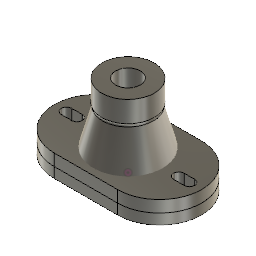
_4&#47;16&#47;19.19b655a6-d3a3-4cc6-afa9-02d68b133b6b (Autodesk Fusion 360 design; units mm, degrees)
Autodesk Fusion 360 part; units mm, degrees
note: some values were not read from the file. Set by a fixed rule: which face or edge a step refers to.
sketch "Sketch1" plane through (0, 0, 0) normal (0, 0, 1) x (1, 0, 0)
  line L0 (27, -36) -> (-27, -36)
  line L1 (-27, 36) -> (27, 36)
  arc A0 (-27, 36) -> (-27, -36) centre (-27, 0) ccw
  arc A1 (27, -36) -> (27, 36) centre (27, 0) ccw
  constraint parallel L0 L1
  constraint horizontal L0
  constraint tangent L1 A0
extrude "Extrude1" add sketch "Sketch1" along normal blind 9 makes body 1
sketch "Sketch2" plane through (0, 0, 9) normal (0, 0, 1) x (-1, 0, 0)
  arc A0 (27, -36) -> (27, 36) centre (27, 0) ccw
  line L0 (27, 36) -> (-27, 36)
  arc A1 (-27, 36) -> (-27, -36) centre (-27, 0) ccw
  line L1 (-27, -36) -> (27, -36)
  line L2 (43.5, -4.5) -> (52.5, -4.5)
  line L3 (52.5, 4.5) -> (43.5, 4.5)
  arc A2 (52.5, -4.5) -> (52.5, 4.5) centre (52.5, 0) ccw
  arc A3 (43.5, 4.5) -> (43.5, -4.5) centre (43.5, 0) ccw
  point P0 (48, 0)
  constraint parallel L2 L3
  constraint horizontal L2
extrude "Extrude2" cut sketch "Sketch2" against normal blind 53 contours L2 L3 A2 A3 bodies 1
sketch "Sketch3" plane through (0, 0, 9) normal (0, 0, 1) x (-1, 0, 0)
  line L0 (52.5, -4.5) -> (43.5, -4.5)
  arc A0 (43.5, 4.5) -> (43.5, -4.5) centre (43.5, 0) ccw
  line L1 (43.5, 4.5) -> (52.5, 4.5)
  arc A1 (52.5, -4.5) -> (52.5, 4.5) centre (52.5, 0) ccw
  arc A2 (27, -36) -> (27, 36) centre (27, 0) ccw
  line L2 (27, 36) -> (-27, 36)
  arc A3 (-27, 36) -> (-27, -36) centre (-27, 0) ccw
  line L3 (-27, -36) -> (27, -36)
  line L4 (-52.5, 4.5) -> (-43.5, 4.5)
  line L5 (-39, 0.0028) -> (-39, -0.0028)
  line L6 (-43.4972, -4.5) -> (-52.5, -4.5)
  arc A4 (-43.5028, -4.5) -> (-43.5, 4.5) centre (-43.5, 0) ccw
  arc A5 (-52.5, 4.5) -> (-52.5, -4.5) centre (-52.5, 0) ccw
  constraint perpendicular L4 L5
  constraint parallel L4 L6
  constraint horizontal L4
  constraint coincident L6 A4.start
  constraint coincident A4 L5.end
  constraint coincident A4 L6.start
  constraint coincident A4 L5.start
extrude "Extrude3" cut sketch "Sketch3" against normal blind 31 contours L4 L5 L6 A4 A5 bodies 1
copy_body "Body->Comp1" bodies 1 removing the originals makes body 2 in component "Component"
sketch "Sketch4" plane through (0, 0, 0) normal (0, 1, 0) x (1, 0, 0)
sketch "Sketch5" plane through (0, 0, 9) normal (0, 0, 1) x (-1, 0, 0)
  line L0 (-52.5, 4.5) -> (-43.5, 4.5)
  arc A0 (-43.5028, -4.5) -> (-43.5, 4.5) centre (-43.5, 0) ccw
  line L1 (-43.5028, -4.5) -> (-52.5, -4.5)
  arc A1 (-52.5, 4.5) -> (-52.5, -4.5) centre (-52.5, 0) ccw
  line L2 (52.5, -4.5) -> (43.5, -4.5)
  arc A2 (43.5, 4.5) -> (43.5, -4.5) centre (43.5, 0) ccw
  line L3 (43.5, 4.5) -> (52.5, 4.5)
  arc A3 (52.5, -4.5) -> (52.5, 4.5) centre (52.5, 0) ccw
  arc A4 (27, -36) -> (27, 36) centre (27, 0) ccw
  line L4 (27, 36) -> (-27, 36)
  arc A5 (-27, 36) -> (-27, -36) centre (-27, 0) ccw
  line L5 (-27, -36) -> (27, -36)
sketch "Sketch6" plane through (0, 0, 0) normal (0, 1, 0) x (1, 0, 0)
  line L0 (-63, -9) -> (-27, -9)
  line L1 (0, -9) -> (-33, -9)
  line L2 (0, -9) -> (0, -52)
  line L3 (0, -52) -> (-21, -52)
  line L4 (-21, -52) -> (-33, -9)
  point P0 (0, -9)
  constraint coincident P0 L1.start
  constraint parallel L0 L1
  constraint perpendicular L1 L2
  constraint perpendicular L2 L3
revolve "Revolve1" add sketch "Sketch6" angle 360 about axis through (0, 0, 9) along (0, 0, 1) bodies 2 in component "Component"
sketch "Sketch7" plane through (0, 0, 0) normal (0, 1, 0) x (1, 0, 0)
  line L0 (27, 0) -> (-27, 0)
  line L1 (0, 0) -> (0, -47)
  line L2 (0, 0) -> (-30, 0)
  line L3 (0, -47) -> (-14.4884, -47)
  line L4 (-27, 0) -> (-14.4884, -47)
  dimension "d27" = 47
  dimension "d28" = 30
  constraint coincident L1.start L2.start
  constraint perpendicular L0 L1
  constraint perpendicular L1 L2
  constraint perpendicular L1 L3
  constraint coincident L0.end L4.start
  constraint coincident L3 L4.end
  measures "d27" distance of L1.start L1.end
  measures "d28" distance of L1.start L2.end
revolve "Revolve2" cut sketch "Sketch7" angle 360 about axis through (0, 0, 0) along (0, 0, 1) bodies 2 in component "Component"
sketch "Sketch8" plane through (0, 0, 52) normal (0, 0, 1) x (-1, 0, 0)
  circle A0 centre (0, 0) radius 21
  circle A1 centre (0, 0) radius 22.5
  dimension "d30" = 45
  constraint concentric A0 A1
  measures "d30" diameter of A1
extrude "Extrude1'" add sketch "Sketch8" along normal blind 18 contours A0 | A1 bodies 2 in component "Component"
sketch "Sketch9" plane through (0, 0, 70) normal (0, 0, 1) x (-1, 0, 0)
  circle A0 centre (0, 0) radius 22.5
  circle A1 centre (0, 0) radius 10.5
  dimension "d33" = 21
  constraint concentric A0 A1
  measures "d33" diameter of A1
extrude "Extrude2'" cut sketch "Sketch9" against normal blind 42 contours A1 bodies 2 in component "Component"
fillet "Fillet1" radius 3 1 edges at (-19.5789, 7.5939, 52) on bodies 2 in component "Component"
fillet "Fillet2" radius 3 1 edges at (30.7668, -11.9333, 9) on bodies 2 in component "Component"
sketch "Sketch10" plane through (0, 0, 9) normal (0, 0, 1) x (-1, 0, 0)
  circle A0 centre (0, 0) radius 16
  dimension "d38" = 32
  constraint coincident A0.centre origin
  measures "d38" diameter of A0
extrude "Extrude4" add sketch "Sketch10" along normal mid plane 24 separate body makes body 3
sketch "Sketch11" plane through (0, 0, 0) normal (0, 1, 0) x (1, 0, 0)
  line L0 (16, 3) -> (-16, 3)
  line L1 (0, 3) -> (-37, 3)
  line L2 (0, 3) -> (0, -51)
  line L3 (-44, -61) -> (-44, -51)
  line L4 (-30, -51) -> (-30, -61)
  arc A0 (-44, -61) -> (-30, -61) centre (-37, -1) ccw
  line L5 (-30, -51) -> (-44, -51)
  dimension "d41" = 37
  dimension "d42" = 54
  constraint midpoint L0 L1.start
  constraint parallel L0 L1
  constraint perpendicular L0 L2
  constraint parallel L3 L4
  constraint perpendicular L3 L5
  measures "d41" distance of L1.start L1.end
  measures "d42" distance of L1.start L2.end
revolve "Revolve1'" add sketch "Sketch11" angle 360 about axis through (-30, 0, 51) along (-1, 0, 0) separate body makes body 4
sketch "Sketch12" plane through (0, 0, 0) normal (0, 1, 0) x (1, 0, 0)
  line L0 (-30, -41) -> (-30, -61)
  line L1 (-37, -41.1323) -> (-37, -50.37)
  line L2 (-37, -50.37) -> (-32, -50.37)
  line L3 (-32, -40.8) -> (-32, -50.37)
  line L4 (-32, -40.8) -> (-17, -18.7213)
  line L5 (-37, -41.1323) -> (-18.646, -14)
  line L6 (-17, -18.7213) -> (0, -18.7213)
  line L7 (16, 3) -> (-16, 3)
  line L8 (0, 3) -> (0, -14)
  line L9 (0, -14) -> (-18.646, -14)
  line L10 (0, -18.7213) -> (0, -14)
  dimension "d52" = 17
  constraint vertical L1
  constraint perpendicular L2 L3
  constraint vertical L3
  constraint horizontal L6
  constraint coincident L7 L8.start
  constraint perpendicular L7 L8
  constraint perpendicular L8 L9
  constraint perpendicular L9 L10
  measures "d52" distance of L8.start L8.end
extrude "Extrude5" add sketch "Sketch12" along normal mid plane 60 bodies 3 4
sketch "Sketch13" plane through (-44, 0, 0) normal (-1, 0, 0) x (0, -1, 0)
  circle A0 centre (0, 51) radius 10
  circle A1 centre (0, 51) radius 5
  dimension "d58" = 10
  constraint concentric A0 A1
  measures "d58" diameter of A1
extrude "Extrude6" cut sketch "Sketch13" against normal blind 120 contours A1 bodies 3
sketch "Sketch14" plane through (0, 0, 0) normal (0, 1, 0) x (1, 0, 0)
  line L0 (16, 3) -> (-16, 3)
  line L1 (-15.4636, 3) -> (-15.4636, 1.5)
  line L2 (-15.4636, 1.5) -> (-35, 1.5)
  line L3 (-44, -41) -> (-44, -61)
  line L4 (-44, -41.5754) -> (-43, -41.5754)
  line L5 (-43, -41.5754) -> (-35, 1.5)
  line L6 (-43, -41.5754) -> (-36, -41)
  line L7 (-36, -41) -> (-34.8709, -37.9849)
  line L8 (-34.8709, -37.9849) -> (-16.9352, -15.6365)
  line L9 (-16.9352, -15.6365) -> (-15.8931, -15.5509)
  line L10 (-15.8931, -15.5509) -> (-15.8931, 1.5)
  line L11 (-18.646, -14) -> (-37, -41.1323)
  dimension "d61" = 1.5
  dimension "d62" = 1
  constraint coincident L0 L1.start
  constraint perpendicular L0 L1
  constraint perpendicular L1 L2
  constraint coincident L3 L4.start
  constraint perpendicular L3 L4
  constraint parallel L6 L9
  constraint coincident L2 L10.end
  constraint perpendicular L2 L10
  constraint coincident L7.end L11
  measures "d61" distance of L1.start L1.end
  measures "d62" distance of L4.start L4.end
extrude "Extrude7" add sketch "Sketch14" along normal mid plane 10 contours L2 L5 L6 L8 L9 L10 L11 bodies 3
mirror "Mirror2" about plane through (0, 0, 0) normal (1, 0, 0) of 22 faces at (-30.2034, 5, 17.8597) (-30.87, 21.6667, 32.0705) (-41.4417, -1.0199, 61.1925) (-33.6667, 16.856, 50.37) (-33.6667, -16.856, 50.37) (-7.7456, 25.1091, 14) (-30.87, -21.6667, 32.0705) (-40.3147, 4.563, 41.3546) (-39.3333, -4.9752, 50.5022) (-11.882, 30, 15.5738) (-37.6236, 0, 12.6263) (-11.882, -30, 15.5738) (-28.6667, 0, -1.5) (-27, -10, 33.4404) (-32, 23.3241, 46.6763) (-37, 23.3389, 46.5598) (-40.3094, -4.5628, 41.3542) (-44, -0.6214, 59.2914) (-30.2034, -5, 17.8597) (-7.7456, -25.1091, 14) (-30, -0.6214, 59.2914) (-37, -23.3965, 46.7953) on bodies 3
fillet "Fillet1'" radius 8 2 edges at (-17, 0, 18.7213) (32, -20.0901, 50.37) on bodies 3
sketch "Sketch15" plane through (0, 0, 21) normal (0, 0, 1) x (-1, 0, 0)
  circle A0 centre (0, 0) radius 16
  circle A1 centre (0, 0) radius 10
  dimension "d67" = 20
  constraint concentric A0 A1
  measures "d67" diameter of A1
extrude "Extrude8" cut sketch "Sketch15" against normal blind 50 contours A1 bodies 3
fillet "Fillet2'" radius 8 1 edges at (-32, 0, 40.8) on bodies 3
fillet "Fillet3" radius 8 1 edges at (17, 0, 18.7213) on bodies 3
sketch "Sketch16" plane through (0, 0, 21) normal (0, 0, 1) x (-1, 0, 0)
  circle A0 centre (0, 0) radius 10
  circle A1 centre (0, 0) radius 16
  circle A2 centre (0, 0) radius 13
  dimension "d72" = 26
  constraint concentric A0 A2
  measures "d72" diameter of A2
extrude "Extrude9" cut sketch "Sketch16" against normal blind 6 contours A2 bodies 3
thread "Thread1" "ISO Metric profile 10.0 M10x1.5 6H" major diameter 10.198 minor diameter 8.526 pitch 1.5 angle 60 resizes the face on face at (-39.3333, -4.9752, 50.5022) on bodies 3
thread "Thread2" "ISO Metric profile 10.0 M10x1.5 6H" major diameter 10.198 minor diameter 8.526 pitch 1.5 angle 60 resizes the face on face at (34.6667, -4.9938, 50.7508) on bodies 3
copy_body "Body->Comp2" bodies 3 removing the originals makes body 5 in component "Component'"
sketch "Sketch17" plane through (0, 0, 9) normal (0, 0, 1) x (-1, 0, 0)
  circle A0 centre (0, 0) radius 20
  dimension "d75" = 40
  constraint coincident A0.centre origin
  measures "d75" diameter of A0
extrude "Extrude10" add sketch "Sketch5" along normal blind 10 separate body makes body 6
extrude "Extrude11" add sketch "Sketch17" along normal mid plane 84 separate body makes body 7
sketch "Sketch18" plane through (0, 0, 51) normal (0, 0, 1) x (-1, 0, 0)
  circle A0 centre (0, 0) radius 20
  circle A1 centre (0, 0) radius 21
  dimension "d80" = 42
  constraint concentric A0 A1
  measures "d80" diameter of A1
extrude "Extrude12" add sketch "Sketch18" along normal blind 6 contours A0 | A1 bodies 7
sketch "Sketch19" plane through (0, 0, -33) normal (0, 0, -1) x (1, 0, 0)
  circle A0 centre (0, 0) radius 20
  circle A1 centre (0, 0) radius 21
  dimension "d83" = 42
  constraint concentric A0 A1
  measures "d83" diameter of A1
extrude "Extrude13" add sketch "Sketch19" along normal blind 6 contours A0 | A1 bodies 7
fillet "Fillet4" radius 2.5 2 edges at (19.5789, 7.5939, 57) (18.6465, 7.2323, 51) on bodies 7
fillet "Fillet5" radius 2.5 2 edges at (18.6465, -7.2323, -33) (-19.5789, 7.5939, -39) on bodies 7
sketch "Sketch20" plane through (0, 0, 57) normal (0, 0, 1) x (-1, 0, 0)
  circle A0 centre (0, 0) radius 18.5
  circle A1 centre (0, 0) radius 12
  dimension "d88" = 24
  constraint concentric A0 A1
  measures "d88" diameter of A1
extrude "Extrude14" cut sketch "Sketch20" against normal blind 120 contours A1 bodies 7
sketch "Sketch21" plane through (0, 0, 0) normal (1, 0, 0) x (0, 1, 0)
  circle A0 centre (0, 0) radius 7.5
  dimension "d91" = 15
  constraint coincident A0.centre origin
  measures "d91" diameter of A0
extrude "Extrude15" add sketch "Sketch21" along normal mid plane 114 bodies 7
copy_body "Body->Comp3" bodies 6 removing the originals makes body 8 in component "Component''"
copy_body "Body->Comp4" bodies 7 removing the originals makes body 9 in component "Component'''"
sketch "Sketch22" plane through (0, 0, 0) normal (0, 0, 1) x (1, 0, 0)
  circle A0 centre (0, 0) radius 20
  circle A1 centre (0, 0) radius 10
  dimension "d94" = 40
  dimension "d95" = 20
  constraint coincident A0.centre A1.centre
  measures "d94" diameter of A0
  measures "d95" diameter of A1
extrude "Extrude16" add sketch "Sketch22" along normal mid plane 32 separate body makes body 10
thread "Thread3" "ISO Metric profile 20.0 M20x2.5 6H" major diameter 20.2925 minor diameter 17.519 pitch 2.5 angle 60 resizes the face on face at (9.9876, -0.4985, 10.6667) on face at (9.9876, -0.4985, -10.6667) on bodies 10
copy_body "Body->Comp5" bodies 10 removing the originals makes body 11 in component "Component''''"
sketch "Sketch23" plane through (0, 0, 0) normal (0, 1, 0) x (1, 0, 0)
  line L0 (-27, 0) -> (27, 0)
  line L1 (20, 0) -> (20, -4)
  line L2 (0, -4) -> (0, -12)
  line L3 (0, -12) -> (-8, -12)
  line L4 (-8, -12) -> (-8, -10)
  line L5 (-8, -10) -> (-16, -10)
  line L6 (0, -4) -> (-16, -4)
  line L7 (-16, -10) -> (-16, -4)
  dimension "d99" = 8
  dimension "d101" = 8
  constraint coincident L0 L1.start
  constraint perpendicular L2 L3
  constraint perpendicular L3 L4
  constraint perpendicular L4 L5
  constraint perpendicular L2 L6
  constraint perpendicular L0 L7
  measures "d99" distance of L2.start L2.end
  measures "d101" distance of L4.end L5.end
revolve "Revolve2'" add sketch "Sketch23" angle 360 about axis through (0, 0, 4) along (-1, 0, 0) separate body makes body 12
component "Component" placed x (1, 0, 0) y (0, 1, 0) z (0, 0, 1) at (0, 0, 0)
component "Component'" placed x (1, 0, 0) y (0, 1, 0) z (0, 0, 1) at (0, 0, 0)
component "Component''" placed x (1, 0, 0) y (0, 1, 0) z (0, 0, 1) at (0, 0, 0)
component "Component'''" placed x (1, 0, 0) y (0, 1, 0) z (0, 0, 1) at (0, 0, 0)
component "Component''''" placed x (1, 0, 0) y (0, 1, 0) z (0, 0, 1) at (0, 0, 0)
